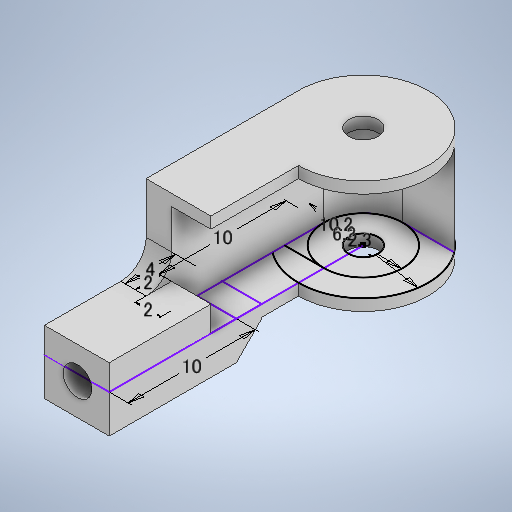
# Autodesk Inventor part: srod2.5_2.25
Saved by Autodesk Inventor 2025 (Build 290162000, 162)
## iProperties
Created: 2024-08-08
Part Number: srod2.5_2.25
Material: 一般
Document SubType Name: Modeling
Designer: Saigusa
Density: 1 g/cm^3
Appearance: 既定
Author: Saigusa
Autodesk Inventor part; units mm, degrees
ref_plane "YZ Plane" through (0, 0, 0) normal (1, 0, 0) x (0, 1, 0)
ref_plane "XZ Plane" through (0, 0, 0) normal (0, 1, 0) x (-1, 0, 0)
ref_plane "XY Plane" through (0, 0, 0) normal (0, 0, 1) x (1, 0, 0)
sketch "スケッチ1" plane through (0, 0, 0) normal (0, 1, 0) x (-1, 0, 0)
  circle A0 centre (0, 0) radius 1.15
  circle A1 centre (0, 0) radius 3.1
  circle A2 centre (0, 0) radius 5.1
  line L0 (3.1, 0) -> (5.1, 0)
  line L1 (5.1, 0) -> (5.1, 10)
  line L2 (5.1, 10) -> (3.1, 10)
  line L3 (3.1, 10) -> (3.1, 0)
  line L4 (0, 3.1) -> (3.1, 3.1)
  line L5 (5.1, 0) -> (1.8843, -2.4616)
  line L6 (5.1, 10) -> (0, 10)
  line L7 (0, 10) -> (0, 20)
  line L8 (0, 20) -> (5.1, 20)
  line L9 (5.1, 20) -> (5.1, 10)
  line L10 (0, 10) -> (0, 0)
  line L11 (0, -3.1) -> (-4.0497, -3.1)
  line L12 (3.1, 10) -> (5.1, 10)
  line L13 (5.1, 10) -> (5.1, 12)
  line L14 (5.1, 12) -> (3.1, 12)
  line L15 (3.1, 12) -> (3.1, 10)
  line L16 (3.1, 12) -> (0, 12)
  line L17 (0, 12) -> (0, 10)
  line L18 (0, 10) -> (3.1, 10)
  line L19 (3.1, 10) -> (3.1, 12)
  line L20 (0, 12) -> (5.1, 12)
  line L21 (5.1, 12) -> (5.1, 8)
  line L22 (5.1, 8) -> (0, 8)
  line L23 (0, 8) -> (0, 12)
  point P0 (0, 5.1)
  dimension "d2" = 10.2
  dimension "d0" = 2.3
  dimension "d1" = 6.2
  dimension "d3" = 10
  dimension "d4" = 10
  dimension "d7" = 2
  dimension "d8" = 2
  dimension "d22" = 4
  constraints: 48 end point, 10 parallel, 7 perpendicular, 5 horizontal, 4 point on circle, 3 coincident, 3 point on line, 2 centre point, 2 tangent, 1 vertical, 3 other
  measures "d0" diameter of A0
  measures "d1" diameter of A1
  measures "d3" distance of L1.end L0.end
  measures "d4" distance of L6.end L7.end
  measures "d7" distance of L14.end L13.end
  measures "d8" distance of L13.end L12.end
  measures "d22" distance of L20.end L21.end
extrude "押し出し1" add sketch "スケッチ1" along normal blind 7.1 contours L0 L5 A1 | L3 A2 L0 | A1 L5 A2 L11 | A2 L3 L22 L1 | L22 L3 L2 L1 | L2 L15 L14 L9
extrude "押し出し2" add sketch "スケッチ1" against normal blind 0.9
sketch "スケッチ2" plane through (0, 7.1, 0) normal (0, 1, 0) x (1, 0, 0)
  circle A0 centre (0, 0) radius 1.15
  circle A1 centre (0, 0) radius 3.1
  circle A2 centre (0, 0) radius 5.1
  line L0 (0, -12) -> (-5.1, -12)
  line L1 (0, 0) -> (-5.1, 0)
  line L2 (-5.1, 0) -> (-5.1, -12)
  line L3 (-5.1, -12) -> (0, -12)
  line L4 (0, -12) -> (0, 0)
  point P0 (0, -5.1)
  dimension "d11" = 2.3
  dimension "d12" = 6.2
  dimension "d13" = 10.2
  dimension "d14" = 5.1
  dimension "d15" = 12
  constraints: 10 end point, 3 centre point, 3 coincident, 2 parallel, 1 horizontal, 1 perpendicular
  measures "d11" diameter of A0
  measures "d12" diameter of A1
  measures "d13" diameter of A2
  measures "d14" distance of L3.end L0.end
  measures "d15" distance of L0.end L1.end
extrude "押し出し3" add sketch "スケッチ2" along normal blind 0.9 contours A0 L1 A1 L4 | A0 L4 A1 L1 | L1 A2 L4 A1 | A1 L4 A2 L1 | A2 L4 L0 L2
extrude "押し出し4" add sketch "スケッチ1" along normal blind 2 contours L7 L8 L9 L14 L16
extrude "押し出し5" add sketch "スケッチ1" against normal blind 3 contours L10 L6 L3 L22 | L22 L3 L2 L1 | L7 L16 L15 L6 | L2 L15 L14 L9 | L7 L8 L9 L14 L16
chamfer "面取り1" distance 2 angle 45 1 edges at (-2.55, -3, 8)
sketch "スケッチ3" plane through (-5.1, 2, 20) normal (0, 0, 1) x (1, 0, 0)
  line L0 (0, -5) -> (0, 0) projected
  line L1 (0, 0) -> (2.6, 0)
  line L2 (2.6, 0) -> (2.6, -2.5)
  line L3 (2.6, -2.5) -> (0, -2.5)
  line L4 (0, -2.5) -> (0, 0)
  circle A0 centre (2.6, -2.5) radius 1.125
  point P0 (5.1, -2)
  dimension "d26" = 2.6
  dimension "d27" = 2.5
  dimension "d28" = 2.25
  constraints: 8 end point, 2 parallel, 1 centre point, 1 coincident, 1 horizontal, 1 perpendicular
  measures "d26" distance of L2.end L3.end
  measures "d27" distance of L1.end L2.end
  measures "d28" diameter of A0
hole "穴1" at (-2.5, -0.5, 20) direction (0, 0, -1) diameter 2.25 depth 7
fillet "フィレット1" radius 2 1 edges at (-4.1, 2, 12)
